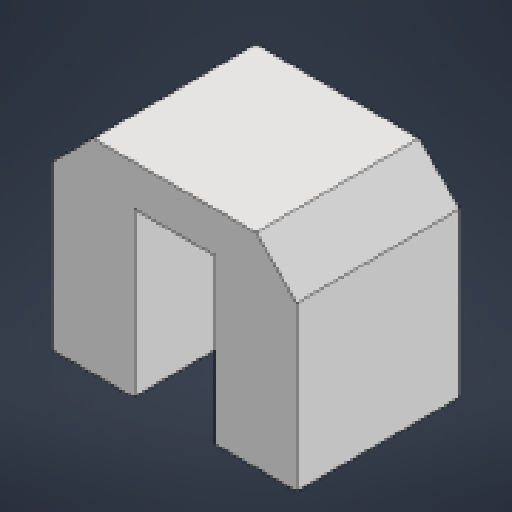
# Autodesk Inventor part: 3DPRINT,WIRE-GUARD,LOOP
Saved by Autodesk Inventor 2026.1 (Build 301233020, 233B)
## iProperties
Created: 2026-03-02
Part Number: 3DPRINT,WIRE-GUARD,LOOP
Material: Generic
Document SubType Name: Modeling
Designer: Owen L
Density: 1 g/cm^3
Appearance: Default
Mass: 0.336063 g
Surface Area: 3.96455 cm^2
Volume: 0.336063 cm^3
Author: Owen L
Autodesk Inventor part; units mm, degrees
ref_plane "YZ Plane" through (0, 0, 0) normal (1, 0, 0) x (0, 1, 0)
ref_plane "XZ Plane" through (0, 0, 0) normal (0, 1, 0) x (-1, 0, 0)
ref_plane "XY Plane" through (0, 0, 0) normal (0, 0, 1) x (1, 0, 0)
sketch "Sketch1" plane through (0, 0, 0) normal (0, 0, 1) x (1, 0, 0)
  line L0 (-4.7625, -6.35) -> (-1.5875, -6.35)
  line L1 (-1.5875, -6.35) -> (-1.5875, 0)
  line L2 (-1.5875, 0) -> (1.5875, 0)
  line L3 (1.5875, 0) -> (1.5875, -6.35)
  line L4 (1.5875, -6.35) -> (4.7625, -6.35)
  line L5 (4.7625, -6.35) -> (4.7625, 1.5875)
  line L6 (4.7625, 1.5875) -> (-4.7625, 1.5875)
  line L7 (-4.7625, 1.5875) -> (-4.7625, -6.35)
  point P0 (0, 0)
  point P1 (0, 0)
  point P2 (0, 1.5875)
  dimension "d0" = 3.175
  dimension "d1" = 3.175
  dimension "d2" = 6.35
  dimension "d3" = 1.5875
  constraints: 16 end point, 6 perpendicular, 2 coincident, 2 midpoint, 2 point on line, 1 horizontal, 1 vertical alignment
  measures "d0" distance of L3.end L4.end
  measures "d1" distance of L1.end L2.end
  measures "d2" distance of L2.end L3.end
  measures "d3" distance between parallel lines of L2 L6
extrude "Extrusion1" add sketch "Sketch1" along normal blind 6.35
chamfer "Chamfer1" distance 1.5875 angle 45 2 edges at (-4.7625, 1.5875, 3.175) (4.7625, 1.5875, 3.175)
body "Solid1"
